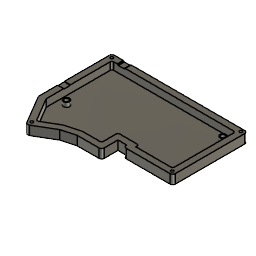
Right_Enclosure (Autodesk Fusion 360 design; units mm, degrees)
part number: 2026-07-18-09-43-34-822
Autodesk Fusion 360 part; units mm, degrees
sketch "Right_enclosure_outline" plane through (0, 0, 0) normal (0, 0, 1) x (1, 0, 0)
  line L0 (-73.4538, 34.3576) -> (65.5462, 34.3576)
  arc A0 (-73.5521, 34.3552) -> (-74.4514, 33.4559) centre (-73.4538, 33.3576) ccw
  line L1 (-74.4538, -39.6424) -> (-74.4538, 33.3576)
  line L2 (-58.9585, -65.7908) -> (-74.4538, -39.6424)
  line L3 (-39.4538, -55.6424) -> (-57.5971, -66.1464)
  line L4 (-21.4538, -50.6424) -> (-39.4538, -55.6424)
  arc A1 (-58.9067, -65.8736) -> (-57.6828, -66.1933) centre (-58.0982, -65.2811) ccw
  line L5 (-0.9538, -50.6424) -> (-21.4538, -50.6424)
  arc A2 (-0.8556, -50.64) -> (0.0438, -49.7406) centre (-0.9538, -49.6424) ccw
  line L6 (0.0462, -32.6424) -> (0.0462, -49.6424)
  line L7 (24.5462, -31.6424) -> (1.0462, -31.6424)
  line L8 (25.5462, -34.6424) -> (25.5462, -32.6424)
  line L9 (64.5462, -35.6424) -> (26.5462, -35.6424)
  line L10 (66.5462, 33.3576) -> (66.5462, -33.6424)
  line L11 (2.5, -32.5) -> (22.5, -32.5)
  line L12 (-56.6719, -66.5254) -> (-39.1, -56.2)
  line L13 (-39.1, -56.2) -> (-21.4538, -51.2983)
  line L14 (-21.4538, -51.2983) -> (-1.5, -51.2983)
  arc A3 (22.5, -32.5) -> (24.5, -34.5) centre (22.5, -34.5) cw
  line L15 (24.5, -34.5) -> (24.5, -36.0424)
  line L16 (-74.8538, 31.6376) -> (-74.8538, 0.3904)
  line L17 (-74.8538, 0.3904) -> (-74.8538, -39.752)
  line L18 (-74.8538, 34) -> (-74.8538, 31.6376)
  line L19 (-74.8538, -39.752) -> (-59.4057, -65.8207)
  line L20 (0.5, -49.2983) -> (0.5, -34.5)
  arc A4 (0.5, -34.5) -> (2.5, -32.5) centre (2.5, -34.5) cw
  line L21 (65.0462, 36) -> (-72.8538, 36)
  line L22 (67.0462, -34.0424) -> (67.0462, 34)
  line L23 (44.5449, -36.0424) -> (65.0462, -36.0424)
  line L24 (24.5, -36.0424) -> (44.5449, -36.0424)
  line L25 (-21.4538, -51.2983) -> (-1.5, -51.2983)
  line L26 (2.5, -32.5) -> (22.5, -32.5)
  line L27 (-74.8538, 34) -> (-74.8538, 31.6376)
  arc A5 (67.0462, 34) -> (65.0462, 36) centre (65.0462, 34) ccw
  line L28 (-39.1, -56.2) -> (-21.4538, -51.2983)
  line L29 (0.5, -49.2983) -> (0.5, -34.5)
  line L30 (65.0462, 36) -> (-72.8538, 36)
  line L31 (67.0462, -34.0424) -> (67.0462, 34)
  arc A6 (-72.8538, 36) -> (-74.8538, 34) centre (-72.8538, 34) ccw
  line L32 (-74.8538, 0.3904) -> (-74.8538, -39.752)
  arc A7 (65.0462, -36.0424) -> (67.0462, -34.0424) centre (65.0462, -34.0424) ccw
  line L33 (-56.6719, -66.5254) -> (-39.1, -56.2)
  line L34 (-74.8538, -39.752) -> (-59.4057, -65.8207)
  line L35 (24.5, -34.5) -> (24.5, -36.0424)
  arc A8 (-59.4057, -65.8207) -> (-56.6719, -66.5254) centre (-57.6851, -64.8011) ccw
  arc A9 (-1.5, -51.2983) -> (0.5, -49.2983) centre (-1.5, -49.2983) ccw
  line L36 (44.5449, -36.0424) -> (65.0462, -36.0424)
  line L37 (-74.8538, 31.6376) -> (-74.8538, 0.3904)
  line L38 (24.5, -36.0424) -> (44.5449, -36.0424)
  line L39 (-20.4997, -58.2983) -> (4.5, -58.2983)
  line L40 (-81.8538, -41.6703) -> (-62.3802, -74.532)
  line L41 (7.5, -55.2983) -> (7.5, -39.5)
  arc A10 (-62.3802, -74.532) -> (-58.2795, -75.5891) centre (-59.7994, -73.0026) ccw
  arc A11 (17.5, -40.0424) -> (20.5, -43.0424) centre (20.5, -40.0424) ccw
  line L42 (7.5, -39.5) -> (17.5, -39.5)
  line L43 (-58.2795, -75.5891) -> (-36.3436, -62.6994)
  line L44 (-81.8538, 31.6376) -> (-81.8538, 0.3904)
  line L45 (-81.8538, 0.3904) -> (-81.8538, -41.6703)
  line L46 (74.0462, -40.0424) -> (74.0462, 40)
  arc A12 (74.0462, 40) -> (71.0462, 43) centre (71.0462, 40) ccw
  line L47 (-36.3436, -62.6994) -> (-20.4997, -58.2983)
  line L48 (44.5449, -43.0424) -> (71.0462, -43.0424)
  arc A13 (-78.8538, 43) -> (-81.8538, 40) centre (-78.8538, 40) ccw
  arc A14 (4.5, -58.2983) -> (7.5, -55.2983) centre (4.5, -55.2983) ccw
  arc A15 (71.0462, -43.0424) -> (74.0462, -40.0424) centre (71.0462, -40.0424) ccw
  line L49 (17.5, -39.5) -> (17.5, -40.0424)
  line L50 (-81.8538, 40) -> (-81.8538, 31.6376)
  line L51 (20.5, -43.0424) -> (44.5449, -43.0424)
  line L52 (71.0462, 43) -> (-78.8538, 43)
  circle A16 centre (-78, 39) radius 1.6
  circle A17 centre (-60, -71) radius 1.6
  circle A18 centre (69.7169, -39.1925) radius 1.6
  circle A19 centre (69.6831, 39.8042) radius 1.6
  circle A20 centre (-65.4538, -25.6424) radius 1.5875
  line L53 (-59.5038, -16.8424) -> (-59.5038, -10.8424)
  line L54 (-65.4038, -16.8424) -> (-65.4038, -10.8424)
  circle A21 centre (60.5462, 28.3576) radius 1.5875
  arc A22 (25.5486, -34.7406) -> (26.4479, -35.64) centre (26.5462, -34.6424) ccw
  arc A23 (25.5438, -32.5441) -> (24.6444, -31.6448) centre (24.5462, -32.6424) ccw
  arc A24 (64.6891, -35.6398) -> (66.5436, -33.7853) centre (64.5462, -33.6424) ccw
  arc A25 (66.5438, 33.4559) -> (65.6444, 34.3552) centre (65.5462, 33.3576) ccw
  arc A26 (-72.8538, 36) -> (-74.8538, 34) centre (-72.8538, 34) ccw
  arc A27 (-59.4057, -65.8207) -> (-56.6719, -66.5254) centre (-57.6851, -64.8011) ccw
  arc A28 (-1.5, -51.2983) -> (0.5, -49.2983) centre (-1.5, -49.2983) ccw
  arc A29 (2.5, -32.5) -> (0.5, -34.5) centre (2.5, -34.5) ccw
  arc A30 (24.5, -34.5) -> (22.5, -32.5) centre (22.5, -34.5) ccw
  arc A31 (65.0462, -36.0424) -> (67.0462, -34.0424) centre (65.0462, -34.0424) ccw
  arc A32 (67.0462, 34) -> (65.0462, 36) centre (65.0462, 34) ccw
  dimension "d1" = 2
  constraint tangent L18 A26
  constraint tangent L21 A26
  constraint tangent L12 A27
  constraint tangent L19 A27
  constraint equal A26 A27
  constraint tangent L14 A28
  constraint tangent L20 A28
  constraint equal A26 A28
  constraint tangent L26 A29
  constraint tangent L29 A29
  constraint equal A26 A29
  constraint tangent L26 A30
  constraint tangent L35 A30
  constraint equal A26 A30
  constraint tangent L22 A31
  constraint tangent L23 A31
  constraint equal A26 A31
  constraint tangent L21 A32
  constraint tangent L22 A32
  constraint equal A26 A32
  measures "d1" radius of A26
extrude "Extrude1" add sketch "Right_enclosure_outline" along normal blind 10.5 contours L39 L40 L41 A10 A11 L42 L43 L44 L45 L46 A12 L47 L48 A13 A14 A15 L49 L50 L51 L52
extrude "Extrude2" add sketch "Right_enclosure_outline" along normal blind 2 contours L11 L12 L13 L14 A3 L15 L16 L17 L18 L19 L20 A4 L21 L22 L23 L24 L25 L26 L27 A5 L28 L29 L30 L31 A6 L32 A7 L33 L34 L35 A8 A9 L36 L37 L38 A26 A27 A28 A29 A30 A31 A32 | A20 | A21
sketch "Sketch2" plane through (0, 0, 0) normal (0, 0, 1) x (1, 0, 0)
  circle A0 centre (69.6831, 39.8042) radius 2.75
  circle A1 centre (69.7169, -39.1925) radius 2.75
  circle A2 centre (-60, -71) radius 2.75
  circle A3 centre (-78, 39) radius 2.75
  point P0 (69.6831, 39.8042)
  point P1 (69.7169, -39.1925)
  point P2 (-60, -71)
  point P3 (-78, 39)
  dimension "d6" = 5.5
  dimension "d9" = 5.5
  dimension "d10" = 5.5
  dimension "d11" = 5.5
  constraint coincident P0 A0.centre
  constraint coincident P1 A1.centre
  constraint coincident P2 A2.centre
  constraint coincident P3 A3.centre
  measures "d6" diameter of A0
  measures "d9" diameter of A1
  measures "d10" diameter of A2
  measures "d11" diameter of A3
extrude "Extrude3" cut sketch "Sketch2" along normal blind 3 contours A0
extrude "Extrude4" cut sketch "Sketch2" along normal blind 3 contours A1 | A2 | A3
sketch "Sketch3" plane through (0, 0, 2) normal (0, 0, 1) x (-1, 0, 0)
  line L0 (-24.5, 34.5) -> (-24.5, 36.0424)
  line L1 (-24.5, 36.0424) -> (-65.0462, 36.0424)
  arc A0 (-65.0462, 36.0424) -> (-67.0462, 34.0424) centre (-65.0462, 34.0424) ccw
  line L2 (-67.0462, 34.0424) -> (-67.0462, -34)
  arc A1 (-67.0462, -34) -> (-65.0462, -36) centre (-65.0462, -34) ccw
  line L3 (-65.0462, -36) -> (72.8538, -36)
  arc A2 (72.8538, -36) -> (74.8538, -34) centre (72.8538, -34) ccw
  line L4 (74.8538, -34) -> (74.8538, 39.752)
  line L5 (74.8538, 39.752) -> (59.4057, 65.8207)
  arc A3 (59.4057, 65.8207) -> (56.6719, 66.5254) centre (57.6851, 64.8011) ccw
  line L6 (56.6719, 66.5254) -> (39.1, 56.2)
  line L7 (39.1, 56.2) -> (21.4538, 51.2983)
  line L8 (21.4538, 51.2983) -> (1.5, 51.2983)
  arc A4 (1.5, 51.2983) -> (-0.5, 49.2983) centre (1.5, 49.2983) ccw
  line L9 (-0.5, 49.2983) -> (-0.5, 34.5)
  arc A5 (-2.5, 32.5) -> (-0.5, 34.5) centre (-2.5, 34.5) ccw
  line L10 (-2.5, 32.5) -> (-22.5, 32.5)
  arc A6 (-24.5, 34.5) -> (-22.5, 32.5) centre (-22.5, 34.5) ccw
  circle A7 centre (65.4538, 25.6424) radius 1.5875
  circle A8 centre (-60.5462, -28.3576) radius 1.5875
  circle A9 centre (65.4538, 25.6424) radius 2.45
  circle A10 centre (65.4538, 25.6424) radius 3.45
  circle A11 centre (-60.5462, -28.3576) radius 2.45
  circle A12 centre (-60.5462, -28.3576) radius 3.45
  point P0 (-60.5462, -28.3576)
  dimension "d14" = 4.9
  dimension "d15" = 1
  dimension "d16" = 4.9
  dimension "d17" = 1
  constraint concentric A7 A9
  constraint coincident P0 A8.centre
  measures "d14" diameter of A9
  measures "d16" diameter of A11
extrude "Extrude5" add sketch "Sketch3" along normal blind 4.9 contours A10 | A12
sketch "swopeniing" plane through (-81.8538, 0, 0) normal (-1, 0, 0) x (0, -1, 0)
  line L0 (-40, 0) -> (41.6703, 0)
  line L1 (41.6703, 10.5) -> (-40, 10.5)
  line L2 (-40, 10.5) -> (-40, 0)
  line L3 (41.6703, 0) -> (41.6703, 10.5)
  line L4 (18.0355, 9.995) -> (18.1755, 9.995)
  arc A0 (13.3155, 9.995) -> (13.6755, 10.355) centre (13.3155, 10.355) ccw
  line L5 (11.8255, 9.995) -> (13.1755, 9.995)
  line L6 (17.6755, 12.195) -> (17.6755, 10.355)
  line L7 (18.1755, 9.995) -> (19.5255, 9.995)
  line L8 (13.6755, 10.355) -> (13.6755, 12.195)
  line L9 (19.5255, 12.895) -> (11.8255, 12.895)
  line L10 (13.6755, 12.195) -> (17.6755, 12.195)
  arc A1 (17.6755, 10.355) -> (18.0355, 9.995) centre (18.0355, 10.355) ccw
  line L11 (11.8255, 12.895) -> (11.8255, 9.995)
  line L12 (19.5255, 9.995) -> (19.5255, 12.895)
  line L13 (13.1755, 9.995) -> (13.3155, 9.995)
  line L14 (18.1255, 9.995) -> (13.2255, 9.995)
extrude "Extrude6" cut sketch "swopeniing" against normal blind 20 contours L1 A0 L5 L8 L11 L13 L14 | L1 L4 L6 L7 A1 L12 L14 | L1 A0 L6 L8 A1 L14
sketch "Niceusbopeninig2" plane through (0, 43, 0) normal (0, 1, 0) x (-1, 0, 0)
  line L0 (-71.0462, 0) -> (78.8538, 0)
  line L1 (-71.0462, 10.5) -> (-71.0462, 0)
  line L2 (78.8538, 10.5) -> (-71.0462, 10.5)
  line L3 (78.8538, 0) -> (78.8538, 10.5)
  line L4 (68.0221, 12.5789) -> (68.2393, 12.4584)
  line L5 (68.2393, 12.4584) -> (68.4202, 12.3136)
  line L6 (68.0221, 9.6111) -> (67.7927, 9.5384)
  line L7 (68.7819, 11.4327) -> (68.7819, 10.7693)
  line L8 (68.4202, 12.3136) -> (68.577, 12.1207)
  line L9 (67.7927, 9.5384) -> (67.5393, 9.5145)
  line L10 (68.7579, 11.6741) -> (68.7819, 11.4327)
  line L11 (67.5393, 9.5145) -> (61.085, 9.5145)
  line L12 (59.8424, 11.4327) -> (59.8664, 11.6741)
  line L13 (60.0473, 10.0696) -> (59.9388, 10.2745)
  line L14 (59.9388, 10.2745) -> (59.8664, 10.5159)
  line L15 (60.3853, 9.7316) -> (60.2041, 9.8767)
  line L16 (60.2041, 9.8767) -> (60.0473, 10.0696)
  line L17 (59.8664, 10.5159) -> (59.8424, 10.7693)
  line L18 (59.8424, 10.7693) -> (59.8424, 11.4327)
  line L19 (59.9388, 11.9152) -> (60.0473, 12.1207)
  line L20 (60.2041, 12.3136) -> (60.3853, 12.4584)
  line L21 (67.5393, 12.6755) -> (67.7927, 12.6513)
  line L22 (61.085, 12.6755) -> (67.5393, 12.6755)
  line L23 (60.3853, 12.4584) -> (60.6025, 12.5789)
  line L24 (67.7927, 12.6513) -> (68.0221, 12.5789)
  line L25 (60.6025, 9.6111) -> (60.3853, 9.7316)
  line L26 (68.2393, 9.7316) -> (68.0221, 9.6111)
  line L27 (61.085, 9.5145) -> (60.8316, 9.5384)
  line L28 (60.6025, 12.5789) -> (60.8316, 12.6513)
  line L29 (60.0473, 12.1207) -> (60.2041, 12.3136)
  line L30 (60.8316, 9.5384) -> (60.6025, 9.6111)
  line L31 (68.6853, 10.2745) -> (68.577, 10.0696)
  line L32 (59.8664, 11.6741) -> (59.9388, 11.9152)
  line L33 (68.6853, 11.9152) -> (68.7579, 11.6741)
  line L34 (68.4202, 9.8767) -> (68.2393, 9.7316)
  line L35 (60.8316, 12.6513) -> (61.085, 12.6755)
  line L36 (68.7819, 10.7693) -> (68.7579, 10.5159)
  line L37 (68.577, 10.0696) -> (68.4202, 9.8767)
  line L38 (68.577, 12.1207) -> (68.6853, 11.9152)
  line L39 (68.7579, 10.5159) -> (68.6853, 10.2745)
extrude "Extrude7" cut sketch "Niceusbopeninig2" against normal blind 68 contours L2 L6 L9 L11 L13 L14 L15 L16 L25 L26 L27 L30 L31 L34 L37 L39
